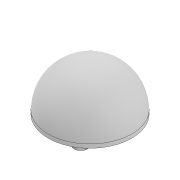
# Autodesk Inventor part: RGB diffuser
Saved by Autodesk Inventor 2020 (Build 240168000, 168)
## iProperties
Created: 2021-12-01
Part Number: RGB diffuser
Material: Generic
Document SubType Name: Modeling
Designer: ferrerx
Density: 1 g/cm^3
Appearance: Default
Author: ferrerx
Autodesk Inventor part; units mm, degrees
ref_plane "YZ Plane" through (0, 0, 0) normal (1, 0, 0) x (0, 1, 0)
ref_plane "XZ Plane" through (0, 0, 0) normal (0, 1, 0) x (-1, 0, 0)
ref_plane "XY Plane" through (0, 0, 0) normal (0, 0, 1) x (1, 0, 0)
sketch "Sketch1" plane through (0, 0, 0) normal (0, 1, 0) x (-1, 0, 0)
  line L0 (-10, 15) -> (10, 15) construction
  line L1 (10, 15) -> (10, -15) construction
  line L2 (10, -15) -> (-10, -15) construction
  line L3 (-10, -15) -> (-10, 15) construction
  line L4 (-10, 15) -> (10, -15) construction
  line L5 (10, 15) -> (-10, -15) construction
  circle A0 centre (10, 15) radius 1.55
  circle A1 centre (10, -15) radius 1.55
  circle A2 centre (-10, -15) radius 1.55
  circle A3 centre (-10, 15) radius 1.55
  circle A4 centre (0, 0) radius 22.5
  line L6 (0, 22.5) -> (0, -22.5)
  dimension "d0" = 20
  dimension "d1" = 30
  dimension "d2" = 3.1
  dimension "d3" = 3.1
  dimension "d4" = 3.1
  dimension "d5" = 3.1
  dimension "d6" = 45
  constraints: 14 end point, 5 centre point, 5 coincident, 2 midpoint, 2 parallel, 2 point on circle, 1 horizontal, 1 perpendicular, 1 vertical
  measures "d0" distance of L1.end L2.end
  measures "d1" distance of L0.end L1.end
  measures "d2" diameter of A1
  measures "d3" diameter of A2
  measures "d4" diameter of A3
  measures "d5" diameter of A0
  measures "d6" diameter of A4
extrude "Extrusion1" add sketch "Sketch1" along normal blind 2
sketch "Sketch2" plane through (0, 2, 0) normal (0, 1, 0) x (1, 0, 0)
  circle A0 centre (0, 0) radius 22.5 projected
  line L0 (0, -22.5) -> (0, 22.5)
  arc A1 (0, 22.5) -> (0, -22.5) centre (0, 0) ccw
  constraints: 4 point on circle, 2 concentric, 2 end point, 1 centre point, 1 vertical
revolve "Revolution1" add sketch "Sketch2" angle 180 about axis through (0, 2, 22.5) along (0, 0, -1) picked at (-6.1724, -4.2605) contours L0 A0
shell "Shell1" thickness 2 removed faces 1 at (-3.0398, 0, -4.5748)
sketch "Sketch4" plane through (0, 0, 0) normal (0, -1, 0) x (1, 0, 0)
  arc A0 (-9.016, -18.4109) -> (-13.527, -15.4036) centre (-10, -15) ccw projected
  circle A1 centre (-10, -15) radius 1.55
  circle A2 centre (-10, -15) radius 1.55 projected
  circle A3 centre (-10, -15) radius 3.55
  circle A4 centre (-10, 15) radius 1.55 projected
  circle A5 centre (-10, 15) radius 1.55
  circle A6 centre (-10, 15) radius 3.55
  arc A7 (9.016, 18.4109) -> (13.527, 15.4036) centre (10, 15) ccw projected
  circle A8 centre (10, 15) radius 1.55
  circle A9 centre (10, 15) radius 1.55 projected
  circle A10 centre (10, 15) radius 3.55
  arc A11 (13.527, -15.4036) -> (9.016, -18.4109) centre (10, -15) ccw projected
  circle A12 centre (10, -15) radius 1.55
  circle A13 centre (10, -15) radius 3.55
  point P0 (0, 0)
  constraints: 8 centre point, 8 coincident, 4 concentric
extrude "Extrusion2" add sketch "Sketch4" along normal blind 2
body "Solid1"
